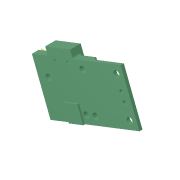
# Autodesk Inventor part: VWheelArmThickRIghtThinSwitchMount
Saved by Autodesk Inventor 2018 (Build 220112000, 112)
## iProperties
Created: 2018-12-14
Part Number: VWheelArmThickRIghtThinSwitchMount
Material: Generic
Document SubType Name: Modeling
Designer: ball
Density: 1 g/cm^3
Appearance: Default
Author: ball
Autodesk Inventor part; units mm, degrees
ref_plane "YZ Plane" through (0, 0, 0) normal (1, 0, 0) x (0, 1, 0)
ref_plane "XZ Plane" through (0, 0, 0) normal (0, 1, 0) x (-1, 0, 0)
sketch "Sketch1" plane through (0, 0, 0) normal (0, 0, 1) x (1, 0, 0)
  circle A0 centre (50.168089, 27.283432) radius 1.778 construction
  circle A1 centre (25.057438, 17.5233) radius 1.778 construction
  circle A2 centre (34.81757, -7.587351) radius 1.778 construction
  circle A3 centre (59.928221, 2.172781) radius 1.778 construction
  circle A4 centre (0, 0) radius 3.5 construction
  circle A5 centre (44.706075, 31.1467) radius 1.778 construction
  circle A6 centre (58.508987, -4.365124) radius 1.778 construction
  circle A7 centre (26.476672, 24.061205) radius 1.778 construction
  circle A8 centre (40.279584, -11.450619) radius 1.778 construction
  line L0 (44.706075, 31.1467) -> (26.476672, 24.061205) construction
  line L1 (58.508987, -4.365124) -> (40.279584, -11.450619) construction
  line L2 (168.541324, -268.17327) -> (30.512209, 86.944969) construction
  circle A9 centre (-14.855389, 15.043191) radius 1.778 construction
  circle A10 centre (1.806199, -27.823373) radius 1.778 construction
  line L3 (67.150197, -1.006416) -> (1.327136, -26.590849)
  line L4 (53.347286, 34.505408) -> (-12.475776, 8.920975)
  line L5 (-12.475776, 8.920975) -> (1.327136, -26.590849)
  circle A11 centre (50.168089, 27.283432) radius 2.2479
  circle A12 centre (59.928221, 2.172781) radius 2.2479
  circle A13 centre (34.81757, -7.587351) radius 2.2479
  circle A14 centre (25.057438, 17.5233) radius 2.2479
  circle A15 centre (0, 0) radius 2.2479
  line L6 (53.347286, 34.505408) -> (67.150197, -1.006416)
  circle A16 centre (27.948918, -10.248098) radius 2.2479
  point P0 (51.216576, 33.677233)
  dimension "d0" = 4.4958
  dimension "d1" = 4.4958
  dimension "d2" = 4.4958
  dimension "d3" = 4.4958
  dimension "d4" = 4.4958
  dimension "d28" = 4.4958
  dimension "d29" = 7.366
  dimension "d30" = 5.57962
  dimension "d31" = 5.588
  constraints: 17 centre point, 14 end point, 5 coincident, 4 point on line, 28 other
  measures "d0" diameter of A11
  measures "d1" diameter of A12
  measures "d2" diameter of A13
  measures "d3" diameter of A14
  measures "d4" diameter of A15
  measures "d28" diameter of A16
  measures "d29" distance of A2.centre A16.centre
  measures "d30" distance from line of L3 A13.centre
  measures "d31" distance from line of L3 A16.centre
extrude "Extrusion1" add sketch "Sketch1" along normal blind 2.286 contours L3 L5 L4 L6 | A16
sketch "Sketch2" plane through (0, 0, 0) normal (0, 0, -1) x (-1, 0, 0)
  line L0 (12.475776, 8.920975) -> (-1.327136, -26.590849)
  line L1 (12.475776, 8.920975) -> (-1.327136, -26.590849)
  line L2 (-1.327136, -26.590849) -> (-43.941324, -10.027355)
  line L3 (-43.941324, -10.027355) -> (-30.138413, 25.484469)
  line L4 (-30.138413, 25.484469) -> (12.475776, 8.920975)
  circle A0 centre (0, 0) radius 2.2479
  circle A1 centre (-34.81757, -7.587351) radius 2.2479
  circle A2 centre (-25.057438, 17.5233) radius 2.2479
  dimension "d7" = 45.72
  constraints: 8 end point, 3 equal length, 1 perpendicular
  measures "d7" distance of L3.end L0.start
extrude "Extrusion2" add sketch "Sketch2" along normal blind 2.794
sketch "Sketch3" plane through (0, 0, -2.794) normal (0, 0, -1) x (-1, 0, 0)
  line L0 (-19.64704, 16.228901) -> (-16.417158, 24.538667) construction
  line L1 (2.38687, 18.02011) -> (-1.109868, 9.023781) construction
  circle A0 centre (-5.05839, 13.167815) radius 1.1938 construction
  circle A1 centre (-13.936346, 16.618543) radius 1.1938 construction
  line L2 (-6.332061, 22.090307) -> (2.025055, 18.842022) construction
  line L3 (-1.109868, 9.023781) -> (-19.64704, 16.228901)
  line L4 (-19.64704, 16.228901) -> (-15.920253, 25.817093)
  line L5 (-15.920253, 25.817093) -> (2.616919, 18.611973)
  line L6 (2.616919, 18.611973) -> (-1.109868, 9.023781)
  circle A2 centre (-13.936346, 16.618543) radius 0.889
  circle A3 centre (-5.05839, 13.167815) radius 0.889
  point P0 (0, 0)
  dimension "d37" = 1.778
  dimension "d38" = 1.778
  constraints: 14 end point, 4 centre point, 2 coincident, 2 parallel, 1 perpendicular, 13 other
  measures "d37" diameter of A2
  measures "d38" diameter of A3
ref_plane "Work Plane1" through (-2.640842, 8.977529, -9.26465) normal (0, 0, 1) x (0.9320689, 0.3622811, 0)
ref_plane "Work Plane2" through (0, 0, -2.794) normal (0, 0, 1) x (1, 0, 0)
sketch "Sketch4" plane through (0, 0, -2.794) normal (0, 0, 1) x (1, 0, 0)
  line L0 (-0.638501, 13.521945) -> (17.898671, 20.727065)
  line L1 (17.898671, 20.727065) -> (-0.638501, 13.521945)
  line L2 (-0.638501, 13.521945) -> (-2.616919, 18.611973)
  line L3 (-2.616919, 18.611973) -> (15.920253, 25.817093)
  line L4 (15.920253, 25.817093) -> (17.898671, 20.727065)
  point P0 (0, 0)
  constraints: 8 end point, 3 equal length, 1 perpendicular
extrude "Extrusion4" add sketch "Sketch4" along normal up to surface (5.08 mm away)
fillet "Fillet1" radius 3.175 1 edges at (37.0399, 7.7286, 0)
sketch "Sketch5" plane through (0, 0, 0) normal (0, 0, -1) x (-1, 0, 0)
  circle A0 centre (-50.168089, 27.283432) radius 2.2479 construction
  circle A1 centre (-59.928221, 2.172781) radius 2.2479 construction
  line L0 (-50.168089, 27.283432) -> (-59.928221, 2.172781) construction
  circle A2 centre (-53.894875, 17.69524) radius 1.524
  circle A3 centre (-56.19536, 11.776603) radius 1.524
  point P0 (0, 0)
  dimension "d15" = 3.048
  dimension "d16" = 3.048
  dimension "d17" = 6.35
  dimension "d18" = 10.287
  constraints: 2 centre point, 2 end point, 2 point on line
  measures "d15" diameter of A2
  measures "d16" diameter of A3
  measures "d17" distance of A3.centre A2.centre
  measures "d18" distance of A2.centre L0.start
extrude "Extrusion5" cut sketch "Sketch5" along normal through all both and the other way through all
sketch "Sketch7" plane through (0, 0, 2.286) normal (0, 0, 1) x (1, 0, 0)
  line L0 (16.123729, -20.839636) -> (11.746293, -9.577467)
  line L1 (1.327136, -26.590849) -> (67.150197, -1.006416)
  line L2 (11.746293, -9.577467) -> (22.470864, -5.408988)
  line L3 (22.470864, -5.408988) -> (26.8483, -16.671157)
  line L4 (-12.475776, 8.920975) -> (1.327136, -26.590849)
  line L5 (16.123729, -20.839636) -> (26.8483, -16.671157)
  line L6 (43.941324, -10.027355) -> (1.327136, -26.590849)
  point P0 (0, 0)
  dimension "d24" = 15.875
  dimension "d25" = 27.3812
  constraints: 8 end point, 2 perpendicular, 1 collinear, 1 point on line
  measures "d24" distance between parallel lines of L4 L0
  measures "d25" distance between parallel lines of L3 L4
extrude "Extrusion6" add sketch "Sketch7" along normal blind 1.27
sketch "Sketch9" plane through (0, 0, -2.794) normal (0, 0, -1) x (-1, 0, 0)
  circle A0 centre (-27.948918, -10.248098) radius 2.2479
  line L0 (-43.941324, -10.027355) -> (-1.327136, -26.590849)
  circle A1 centre (-34.81757, -7.587351) radius 2.2479
  point P0 (0, 0)
  dimension "d32" = 4.4958
  dimension "d33" = 5.588
  dimension "d34" = 7.366
  constraints: 1 centre point
  measures "d32" diameter of A0
  measures "d33" distance from line of L0 A0.centre
  measures "d34" distance of A0.centre A1.centre
extrude "Extrusion7" cut sketch "Sketch9" against normal through all contours A0
extrude "Extrusion8" add sketch "Sketch3" along normal blind 2.667
sketch "Sketch11" plane through (0, 0, -5.461) normal (0, 0, -1) x (-1, 0, 0)
  circle A0 centre (-13.936346, 16.618543) radius 0.889
  circle A1 centre (-13.936346, 16.618543) radius 0.889
  circle A2 centre (-5.05839, 13.167815) radius 0.889
  circle A3 centre (-5.05839, 13.167815) radius 0.889
  point P0 (0, 0)
  constraints: 2 centre point, 2 coincident
hole "Hole1" at (13.936346, 16.618543, -5.461) at (5.05839, 13.167815, -5.461) direction (0, 0, 1) diameter 1.778 end through all
fillet "Fillet4" radius 1.27 5 edges at (18.7729, 18.478, -2.794) (17.8987, 20.7271, -0.254) (10.3785, 12.6263, -2.794) (0.2357, 11.2729, -2.794) (-0.6385, 13.5219, -0.254)
body "Solid1"
